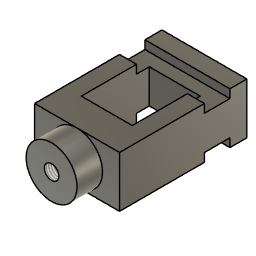
Excercise-2 by chaitanya sharma_ (Autodesk Fusion 360 design; units mm, degrees)
Autodesk Fusion 360 part; units mm, degrees
sketch "Sketch1" plane through (0, 0, 0) normal (0, 1, 0) x (1, 0, 0)
  line L0 (30, 18) -> (-30, 18)
  line L1 (-30, 18) -> (-30, -18)
  line L2 (-30, -18) -> (30, -18)
  line L3 (30, -18) -> (30, 18)
  constraint horizontal L0
  constraint perpendicular L0 L1
  constraint parallel L0 L2
  constraint parallel L1 L3
extrude "Extrude1" add sketch "Sketch1" along normal blind 90
sketch "Sketch2" plane through (0, 0, 0) normal (0, -1, 0) x (1, 0, 0)
  line L0 (30, -18) -> (30, 18)
  line L1 (30, 18) -> (-30, 18)
  line L2 (-30, 18) -> (-30, -18)
  line L3 (-30, -18) -> (30, -18)
  circle A0 centre (0, 0) radius 18
  circle A1 centre (0, 0) radius 6
  dimension "d5" = 12
  constraint coincident A0.centre A1.centre
  constraint concentric A0 A1
  measures "d5" diameter of A1
extrude "Extrude2" add sketch "Sketch2" along normal blind 18 contours A0
thread "Thread1" "ISO Metric profile 12.0 M12x1.75 6H" major diameter 12.2265 minor diameter 10.2735 pitch 1.75 angle 60 resizes the face on face at (5.9925, -12, -0.2991)
sketch "Sketch3" plane through (-30, 0, 0) normal (-1, 0, 0) x (0, -1, 0)
  line L0 (0, -18) -> (0, 18)
  line L1 (0, 18) -> (-90, 18)
  line L2 (-90, 18) -> (-90, -18)
  line L3 (-90, -18) -> (0, -18)
  line L4 (-78, -18) -> (-60, -18)
  line L5 (-60, -18) -> (-60, -12)
  line L6 (-60, -12) -> (-78, -12)
  line L7 (-78, -12) -> (-78, -18)
  constraint horizontal L4
  constraint vertical L5
  constraint horizontal L6
  constraint vertical L7
  constraint coincident L3 L4.start
extrude "Extrude3" cut sketch "Sketch3" against normal blind 60 contours L3 L4 L5 L6 L7
sketch "Sketch4" plane through (-30, 0, 0) normal (-1, 0, 0) x (0, -1, 0)
  line L0 (-78, -18) -> (-78, -12)
  line L1 (-78, -12) -> (-60, -12)
  line L2 (-60, -12) -> (-60, -18)
  line L3 (-60, -18) -> (0, -18)
  line L4 (0, -18) -> (0, 18)
  line L5 (0, 18) -> (-90, 18)
  line L6 (-90, 18) -> (-90, -18)
  line L7 (-90, -18) -> (-78, -18)
  line L8 (-78, 18) -> (-60, 18)
  line L9 (-60, 18) -> (-60, 12)
  line L10 (-60, 12) -> (-78, 12)
  line L11 (-78, 12) -> (-78, 18)
  constraint horizontal L8
  constraint vertical L9
  constraint horizontal L10
  constraint vertical L11
  constraint coincident L5 L8.start
extrude "Extrude4" cut sketch "Sketch4" against normal blind 60 contours L5 L8 L9 L10 L11
sketch "Sketch5" plane through (0, 0, 18) normal (0, 0, 1) x (-1, 0, 0)
  line L0 (-30, -60) -> (30, -60)
  line L1 (30, -60) -> (30, 0)
  line L2 (30, 0) -> (0, 0)
  line L3 (0, 0) -> (-30, 0)
  line L4 (-30, 0) -> (-30, -60)
  line L5 (-30, 0) -> (-30, -21)
  line L6 (-18, -21) -> (-18, -69)
  line L7 (-18, -69) -> (18, -69)
  line L8 (18, -69) -> (18, -21)
  line L9 (18, -21) -> (-18, -21)
  dimension "d21" = 12
  dimension "d22" = 48
  dimension "d23" = 36
  constraint coincident L3.end L4.start
  constraint perpendicular L3 L5
  constraint perpendicular L6 L7
  constraint perpendicular L7 L8
  constraint perpendicular L6 L9
  measures "d21" distance of L5.end L6.start
  measures "d22" distance of L6.start L6.end
  measures "d23" distance of L6.end L7.end
extrude "Extrude5" cut sketch "Sketch5" against normal blind 36 contours L0 L6 L8 L9 | L0 L6 L7 L8
